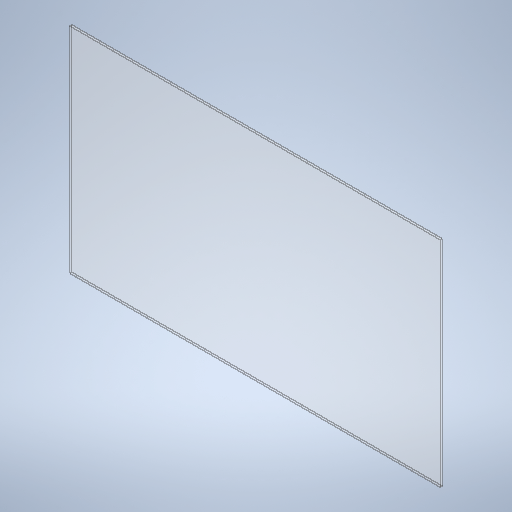
# Autodesk Inventor part: PLANCHA DE CRISTAL TRANSPARENTE 1033x597
Saved by Autodesk Inventor 2025 (Build 290162000, 162)
## iProperties
Created: 2026-02-16
Part Number: PLANCHA DE CRISTAL TRANSPARENTE 1033x597
Material: Cristal
Document SubType Name: Modeling
Designer: Frank
Density: 2.18 g/cm^3
Appearance: Transparente - Claro
Author: Frank
Autodesk Inventor part; units mm, degrees
ref_plane "YZ Plane" through (0, 0, 0) normal (1, 0, 0) x (0, 1, 0)
ref_plane "XZ Plane" through (0, 0, 0) normal (0, 1, 0) x (-1, 0, 0)
ref_plane "XY Plane" through (0, 0, 0) normal (0, 0, 1) x (1, 0, 0)
sketch "Boceto1" plane through (0, 0, 0) normal (0, 0, 1) x (1, 0, 0)
  line L0 (-1033.4, 597.4) -> (0, 597.4)
  line L1 (0, 597.4) -> (0, 0)
  line L2 (0, 0) -> (-1033.4, 0)
  line L3 (-1033.4, 0) -> (-1033.4, 597.4)
  point P0 (0, 0)
  dimension "d2" = 1033.4
  dimension "d3" = 597.4
  constraints: 8 end point, 2 parallel, 2 point on line, 1 horizontal, 1 perpendicular
  measures "d2" distance of L0.start L0.end
  measures "d3" distance of L2.end L0.start
extrude "Extrusión1" add sketch "Boceto1" along normal blind 6
